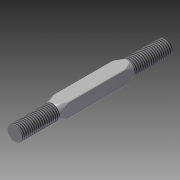
# Autodesk Inventor part: Pieza1
Saved by Autodesk Inventor 2013 (Build 170138000, 138)
## iProperties
Created: 2013-06-07
Part Number: Pieza1
Material: Acero
Document SubType Name: Modeling
Designer: BRAYAN
Density: 1 g/cm^3
Author: BRAYAN
Autodesk Inventor part; units mm, degrees
ref_plane "YZ Plane" through (0, 0, 0) normal (1, 0, 0) x (0, 1, 0)
ref_plane "XY Plane" through (0, 0, 0) normal (0, 0, 1) x (1, 0, 0)
sketch "Boceto1" plane through (0, 0, 0) normal (0, 1, 0) x (-1, 0, 0)
  circle A0 centre (0, 0) radius 3.5
  dimension "d0" = 7
  constraints: 1 centre point, 1 coincident
  measures "d0" diameter of A0
extrude "Extrusión1" add sketch "Boceto1" along normal blind 72
ref_plane "Plano de trabajo1" through (0, 18, 0) normal (0, 1, 0) x (-1, 0, 0)
sketch "Boceto3" plane through (0, 18, 0) normal (0, 1, 0) x (-1, 0, 0)
  line L0 (-3.5, 0) -> (-3.5, -3.5)
  line L1 (-3.5, -3.5) -> (0, -3.5)
  line L2 (-3.5, -3.5) -> (3.5, -3.5)
  line L3 (3.5, -3.5) -> (3.5, 3.5)
  line L4 (3.5, 3.5) -> (-3.5, 3.5)
  line L5 (-3.5, 3.5) -> (-3.5, -3.5)
  point P0 (0, 0)
  dimension "d26" = 3.5
  dimension "d27" = 3.5
  dimension "d28" = 7
  dimension "d29" = 7
  constraints: 12 end point, 2 parallel, 1 horizontal, 1 perpendicular
  measures "d26" distance of L1.end L0.end
  measures "d27" distance of L0.end L0.start
  measures "d28" distance of L4.end L3.end
  measures "d29" distance of L3.end L2.end
extrude "Extrusión3" add sketch "Boceto3" along normal blind 36
sketch "Boceto4" plane through (0, 0, 0) normal (1, 0, 0) x (0, 1, 0)
  line L0 (0, 0) -> (18, 0)
  line L1 (18, 0) -> (18, 3.5)
  line L2 (23, 5) -> (18, 3.5)
  line L3 (18, 0) -> (54, 0)
  line L4 (54, 0) -> (54, 3.5)
  line L5 (49, 5) -> (54, 3.5)
  line L6 (23, 5) -> (24.5315, 10.105)
  line L7 (24.5315, 10.105) -> (47.4685, 10.105)
  line L8 (18, 3.5) -> (7.2687, 12.5016)
  line L9 (7.2687, 12.5016) -> (61.5507, 12.5016)
  line L10 (61.5507, 12.5016) -> (54, 3.5)
  line L11 (49, 5) -> (47.4685, 10.105)
  dimension "d31" = 18
  dimension "d32" = 3.5
  dimension "d36" = 3.5
  constraints: 24 end point, 6 perpendicular, 1 horizontal, 1 parallel
  measures "d31" distance of L0.start L0.end
  measures "d32" distance of L0.end L1.end
  measures "d36" distance of L3.end L4.end
revolve "Revolución2" cut sketch "Boceto4" angle 360 about axis through (0, 0, 0) along (0, 1, 0) contours L8 L9 L10 L5 L11 L7 L6 L2
fillet "Empalme1" radius 0.5 4 edges at (3.5, 36, 3.5) (-3.5, 36, 3.5) (3.5, 36, -3.5) (-3.5, 36, -3.5)
thread "Rosca1" size "M7x1" class "6g" standard "ANSI Metric M Profile" full length
thread "Rosca2" size "M7x1" class "6g" standard "ANSI Metric M Profile" full length
